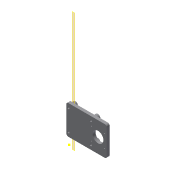
# Autodesk Inventor part: Neje_slide_y_20mmrod_upperplate
Saved by Autodesk Inventor 2019.4 (Build 234330000, 330)
## iProperties
Created: 2021-08-20
Part Number: Neje_slide_y_20mmrod_upperplate
Material: Generic
Document SubType Name: Modeling
Designer: diederichbenedict
Density: 1 g/cm^3
Appearance: Default
Mass: 58.4747 g
Surface Area: 206.633 cm^2
Volume: 58.4747 cm^3
Author: diederichbenedict
Autodesk Inventor part; units mm, degrees
ref_plane "YZ Plane" through (0, 0, 0) normal (1, 0, 0) x (0, 1, 0)
ref_plane "XZ Plane" through (0, 0, 0) normal (0, 1, 0) x (-1, 0, 0)
ref_plane "XY Plane" through (0, 0, 0) normal (0, 0, 1) x (1, 0, 0)
ref_plane "Work Plane1" through (0, 0, 0) normal (0, 0, 1) x (1, 0, 0)
sketch "Sketch1" plane through (0, 0, 0) normal (0, 0, 1) x (1, 0, 0)
  line L0 (40, 0) -> (34, 0) projected
  line L1 (40, 0) -> (40, 260) projected
  line L2 (40, 260) -> (34, 260) projected
  line L3 (34, 0) -> (34, 260) projected
  line L4 (0, 0) -> (6, 0) projected
  line L5 (6, 0) -> (6, 260) projected
  line L6 (0, 260) -> (6, 260) projected
  line L7 (0, 0) -> (0, 260) projected
  line L8 (90, 15.4736) -> (-7, 15.4736)
  line L9 (-7, 15.4736) -> (-7, 85.4736)
  line L10 (-7, 85.4736) -> (90, 85.4736)
  line L11 (90, 85.4736) -> (90, 15.4736)
  line L12 (90, 85.4736) -> (-7, 15.4736) construction
  line L13 (90, 15.4736) -> (-7, 85.4736) construction
  line L14 (14, 0) -> (26, 0) construction
  line L15 (26, 0) -> (26, 260) construction
  line L16 (14, 260) -> (26, 260) construction
  line L17 (14, 0) -> (14, 260) construction
  circle A0 centre (-2, 25.4736) radius 2.45
  circle A1 centre (-2, 75.4736) radius 2.45
  circle A2 centre (51.5, 75.4736) radius 2.45
  circle A3 centre (51.5, 25.4736) radius 2.45
  line L18 (40, 40.4736) -> (-160, 40.4736) projected
  line L19 (40, 60.4736) -> (-160, 60.4736) projected
  line L20 (44.75, 134.6251) -> (44.75, -65.3749)
  line L21 (8.75, 134.6251) -> (8.75, -65.3749)
  line L22 (4.75, 134.6251) -> (4.75, -65.3749)
  dimension "d0" = 50
  dimension "d1" = 7
  dimension "d2" = 70
  dimension "d3" = 4.9
  dimension "d4" = 4.9
  dimension "d5" = 4.9
  dimension "d6" = 4.9
  dimension "d7" = 10
  dimension "d8" = 10
  dimension "d9" = 10
  dimension "d10" = 10
  dimension "d17" = 25
  dimension "d20" = 0
  dimension "d48" = 0
  dimension "d52" = 6.75
  dimension "d54" = 6.75
  constraints: 18 end point, 4 centre point, 3 vertical, 2 parallel, 1 horizontal, 1 perpendicular, 6 other
  measures "d0" distance between parallel lines of L11 L1
  measures "d1" distance between parallel lines of L9 L7
  measures "d2" distance between parallel lines of L10 L8
  measures "d3" diameter of A0
  measures "d4" diameter of A1
  measures "d5" diameter of A2
  measures "d6" diameter of A3
  measures "d7" distance from line of A3.centre L8
  measures "d8" distance from line of A0.centre L8
  measures "d9" distance from line of A1.centre L10
  measures "d10" distance from line of A2.centre L10
  measures "d17" distance between parallel lines of L18 L8
  measures "d20" horizontal distance of A2.centre A3.centre
  measures "d48" horizontal distance of A0.centre A1.centre
  measures "d52" distance from line of A2.centre L20
  measures "d54" distance from line of L22 A1.centre
extrude "Extrusion1" add sketch "Sketch1" along normal blind 7 contours L8 L3 L18 L1 | L1 L10 L20 L8 | L8 L21 L18 L3 | L18 L3 L19 L1 | L20 L10 L11 L8 | L18 L21 L19 L3 | L8 L5 L18 L21 | L19 L3 L10 L1 | L19 L21 L10 L3 | L18 L5 L19 L21 | L8 L22 L18 L5 | L19 L5 L10 L21 | L18 L22 L19 L5 | L8 L7 A0 L18 L22 | L19 L22 L10 L5 | L18 L7 L19 L22 | L8 L9 L18 L7 A0 | L19 L7 A1 L10 L22 | L18 L9 L19 L7 | L19 L9 L10 L7 A1
sketch "Sketch2" plane through (0, 0, 7) normal (0, 0, 1) x (1, 0, 0)
  circle A0 centre (69, 50.4736) radius 9.2 projected
  circle A1 centre (84.5, 34.9736) radius 3 construction
  circle A2 centre (53.5, 34.9736) radius 3 construction
  circle A3 centre (53.5, 65.9736) radius 3 construction
  line L0 (89.5, 67.2664) -> (89.5, 33.6807) projected
  arc A4 (89.5, 67.2664) -> (85.7929, 70.9736) centre (69, 50.4736) ccw projected
  line L1 (52.2071, 70.9736) -> (85.7929, 70.9736) projected
  arc A5 (52.2071, 70.9736) -> (48.5, 67.2664) centre (69, 50.4736) ccw projected
  line L2 (48.5, 33.6807) -> (48.5, 67.2664) projected
  arc A6 (48.5, 33.6807) -> (52.2071, 29.9736) centre (69, 50.4736) ccw projected
  line L3 (85.7929, 29.9736) -> (52.2071, 29.9736) projected
  arc A7 (85.7929, 29.9736) -> (89.5, 33.6807) centre (69, 50.4736) ccw projected
  circle A8 centre (84.5, 34.9736) radius 3 projected
  circle A9 centre (53.5, 34.9736) radius 3 projected
  circle A10 centre (84.5, 65.9736) radius 3 construction
  circle A11 centre (69, 50.4736) radius 4 projected
  circle A12 centre (53.5, 65.9736) radius 3 projected
  circle A13 centre (84.5, 65.9736) radius 1.45
  circle A14 centre (53.5, 65.9736) radius 1.45
  circle A15 centre (53.5, 34.9736) radius 1.45
  circle A16 centre (84.5, 34.9736) radius 1.45
  circle A17 centre (69, 50.4736) radius 12.9144
  point P0 (0, 0)
  dimension "d56" = 2.9
  dimension "d57" = 2.9
  dimension "d58" = 2.9
  dimension "d59" = 2.9
  constraints: 5 centre point, 4 coincident
  measures "d56" diameter of A13
  measures "d57" diameter of A14
  measures "d58" diameter of A15
  measures "d59" diameter of A16
extrude "Extrusion2" cut sketch "Sketch2" against normal through all contours A0 | A11 | A13 | A14 | A15 | A16 | A17
sketch "Sketch3" plane through (0, 0, 7) normal (0, 0, 1) x (1, 0, 0)
  point P0 (0, 0)
fillet "Fillet1" radius 5 4 edges at (90, 85.4736, 3.5) (-7, 85.4736, 3.5) (-7, 15.4736, 3.5) (90, 15.4736, 3.5)
sketch "Sketch6" plane through (0, 0, 0) normal (0, 0, -1) x (-1, 0, 0)
  circle A0 centre (2, 25.4736) radius 2.45 projected
  circle A1 centre (2, 75.4736) radius 2.45 projected
  circle A2 centre (2, 25.4736) radius 5.45
  circle A3 centre (2, 75.4736) radius 5.45
  circle A4 centre (-51.5, 25.4736) radius 6
  circle A5 centre (-51.5, 75.4736) radius 6
  circle A6 centre (-51.5, 75.4736) radius 2.45
  circle A7 centre (-51.5, 25.4736) radius 2.45
  point P0 (0, 0)
  dimension "d42" = 3
  dimension "d43" = 3
  dimension "d55" = 12
  constraints: 6 centre point, 6 other
  measures "d42" radial gap between concentric circles of A0 A2
  measures "d43" radial gap between concentric circles of A1 A3
  measures "d55" diameter of A5
extrude "Extrusion4" add sketch "Sketch6" along normal blind 10
chamfer "Chamfer1" distance 4 angle 45 4 edges at (57.5, 25.4736, 0) (3.45, 25.4736, 0) (57.5, 75.4736, 0) (3.45, 75.4736, 0)
equation "\"d3\" = d6"
equation "\"d4\" = d6"
equation "\"d5\" = d6"
equation "\"d42\" = d45"
equation "\"d43\" = d45"
equation "\"d45\" = 3"
body "Solid1"
